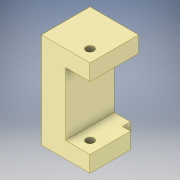
# Autodesk Inventor part: Bauteil2
Saved by Autodesk Inventor 2018.3 (Build 223285000, 285)
## iProperties
Created: 2021-01-25
Part Number: Bauteil2
Material: Nylon 6
Document SubType Name: Modeling
Designer: stege
Density: 1.12 g/cm^3
Appearance: Nylon 6
Author: stege
Autodesk Inventor part; units mm, degrees
ref_plane "YZ Plane" through (0, 0, 0) normal (1, 0, 0) x (0, 1, 0)
ref_plane "XZ Plane" through (0, 0, 0) normal (0, 1, 0) x (-1, 0, 0)
ref_plane "XY Plane" through (0, 0, 0) normal (0, 0, 1) x (1, 0, 0)
sketch "Skizze1" plane through (0, 0, 0) normal (0, 1, 0) x (-1, 0, 0)
  line L0 (3.7731, -4.4076) -> (3.7731, -12.4076)
  line L1 (10.7449, 21.0924) -> (18.7731, 21.0924)
  line L2 (18.7731, 21.0924) -> (18.7731, -37.9076)
  line L3 (18.7731, -37.9076) -> (10.7449, -37.9076)
  line L4 (10.7449, 21.0924) -> (-11.2269, 21.0924)
  line L5 (-11.2269, 21.0924) -> (-11.2269, 11.0924)
  line L6 (-11.2269, 11.0924) -> (3.7731, 11.0924)
  line L7 (10.7449, -37.9076) -> (-11.2269, -37.9076)
  line L8 (-11.2269, -37.9076) -> (-11.2269, -27.9076)
  line L9 (-11.2269, -27.9076) -> (3.7731, -27.9076)
  line L10 (3.7731, -12.4076) -> (3.7731, -12.4076)
  line L11 (3.7731, -4.4076) -> (3.7731, -4.4076)
  line L12 (3.7731, -27.9076) -> (3.7731, -12.4076)
  line L13 (3.7731, -4.4076) -> (3.7731, 11.0924)
  point P0 (0, 0)
  dimension "d1" = 15
  dimension "d2" = 15.5
  dimension "d3" = 15.5
  dimension "d5" = 10
  dimension "d6" = 59
  dimension "d7" = 0
  dimension "d8" = 15
  dimension "d64" = 8
  dimension "d65" = 10
  constraints: 28 end point, 6 parallel, 4 horizontal, 3 perpendicular, 1 point on line
  measures "d1" distance between parallel lines of L5 L13
  measures "d2" distance between parallel lines of L11 L6
  measures "d3" distance between parallel lines of L9 L10
  measures "d5" distance between parallel lines of L4 L6
  measures "d6" distance between parallel lines of L3 L1
  measures "d7" distance between parallel lines of L0 L13
  measures "d8" distance between parallel lines of L13 L2
  measures "d64" distance of L0.start L0.end
  measures "d65" distance between parallel lines of L7 L9
extrude "Extrusion1" add sketch "Skizze1" along normal blind 30
sketch "Skizze2" plane through (0, 30, 0) normal (0, 1, 0) x (1, 0, 0)
  line L0 (11.2269, 27.9076) -> (11.2269, 37.9076) projected
  line L1 (11.2269, 37.9076) -> (6.2269, 37.9076)
  line L2 (6.2269, 37.9076) -> (6.2269, 27.9076)
  line L3 (6.2269, 27.9076) -> (11.2269, 27.9076)
  line L4 (11.2269, 27.9076) -> (11.2269, 37.9076)
  line L5 (-3.7731, 27.9076) -> (11.2269, 27.9076) projected
  point P0 (0, 0)
  dimension "d11" = 0
  dimension "d12" = 5
  constraints: 8 end point, 2 parallel, 1 horizontal, 1 perpendicular
  measures "d11" distance between parallel lines of L5 L3
  measures "d12" distance between parallel lines of L0 L2
extrude "Extrusion2" cut sketch "Skizze2" against normal blind 5
sketch "Skizze6" plane through (-18.7731, 0, 21.0924) normal (0, 0, 1) x (1, 0, 0)
  circle A0 centre (22.5, 7.5) radius 4.6596
  line L0 (30, 0) -> (0, 0) projected
  line L1 (30, 0) -> (30, 30) projected
  point P0 (18.7731, 0)
  dimension "d27" = 7.5
  dimension "d28" = 7.5
  constraints: 1 centre point
  measures "d27" distance from line of L0 A0.centre
  measures "d28" distance from line of L1 A0.centre
hole "Bohrung1" at (3.7269, 7.5, 21.0924) direction (0, 0, -1) diameter 4.917 depth 17 tip angle 118 thread size "M6x1" class "6H" standard "ANSI Metric M Profile"
sketch "Skizze8" plane through (11.2269, 0, -37.9076) normal (0, 0, -1) x (-1, 0, 0)
  circle A0 centre (7.5, 7.5) radius 1.9257
  line L0 (30, 0) -> (0, 0) projected
  line L1 (0, 0) -> (0, 25) projected
  point P0 (11.2269, 0)
  dimension "d45" = 7.5
  dimension "d46" = 7.5
  constraints: 1 centre point
  measures "d45" distance from line of L0 A0.centre
  measures "d46" distance from line of L1 A0.centre
hole "Bohrung3" at (3.7269, 7.5, -37.9076) direction (0, 0, 1) diameter 4.917 depth 17 tip angle 118 thread size "M6x1" class "6H" standard "ANSI Metric M Profile"
